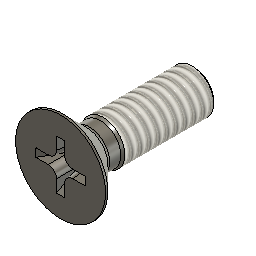
Poker Trophy (Assembly) (Autodesk Fusion 360 archive; units mm, degrees)
design "Countersunk Screw JIS B 1111 - M2x6 H Steel 4.6 Plain"
description: Countersunk Screw JIS B 1111 - M2x6 H
part number: CS JIS B 1111 - M2x6 - H Steel 4.6 Plain
Autodesk Fusion 360 part; units mm, degrees
sketch "Sketch1" plane through (0, 0, 0) normal (0, 1, 0) x (1, 0, 0)
  line L0 (0, -2.1) -> (-2, -2.1)
  line L1 (-2, -2.1) -> (-2, -2)
  line L2 (-2, -2) -> (-0.9, -0.9)
  line L3 (-1, -0.15) -> (-1, 3.9)
  line L4 (-1, 3.9) -> (0, 3.9)
  line L5 (0, 3.9) -> (0, -2.1)
  line L6 (-0.9, -0.3232) -> (-0.9, -0.9)
  line L7 (-1, -0.15) -> (-0.9, -0.3232)
  dimension "d9" = 2
  dimension "d11" = 4
  dimension "d71" = 1.2
  dimension "d72" = 1.8
  dimension "d89" = 4.05
  dimension "d101" = 30
  dimension "d115" = 6
  dimension "d121" = 45
  constraint perpendicular L0 L1
  constraint vertical L3
  constraint perpendicular L3 L4
  constraint perpendicular L0 L5
  constraint collinear origin L0.start L4.end
  constraint horizontal L0
  constraint coincident L2.end L6.end
  constraint coincident L6 L7.end
  constraint coincident L6.start L7.end
  constraint coincident origin L2
  measures "d71" distance of L0 L2.end
  measures "d89" distance of L4 L3.start
  measures "d101" angle of L3 L7
  measures "d115" distance of L0.start L4
  measures "d121" angle of L2 L5
revolve "Revolve1" add sketch "Sketch1" angle 360 about axis through (0, 0, -3.9) along (0, 0, 1) makes body 1
sketch "Sketch2" plane through (0, 0, 2.1) normal (0, 0, 1) x (1, 0, 0)
  line L0 (-0.1833, 0.1833) -> (-1.1, 0.1833)
  line L1 (-1.1, 0.1833) -> (-1.1, -0.1833)
  line L2 (-1.1, -0.1833) -> (-0.1833, -0.1833)
  line L3 (0.1833, -1.1) -> (0.1833, -0.1833)
  line L4 (-0.1833, -1.1) -> (0.1833, -1.1)
  line L5 (-0.1833, -0.1833) -> (-0.1833, -1.1)
  line L6 (1.1, 0.1833) -> (0.1833, 0.1833)
  line L7 (1.1, -0.1833) -> (1.1, 0.1833)
  line L8 (0.1833, -0.1833) -> (1.1, -0.1833)
  line L9 (-0.1833, 1.1) -> (-0.1833, 0.1833)
  line L10 (0.1833, 1.1) -> (-0.1833, 1.1)
  line L11 (0.1833, 0.1833) -> (0.1833, 1.1)
  dimension "d111" = 360
  dimension "d117" = 2.2
  dimension "d122" = 0.3667
  constraint horizontal L0
  constraint perpendicular L0 L1
  constraint vertical L0.start L2.end
  constraint coincident L0.start L9.end
  measures "d117" distance of L4.start L10
  measures "d122" distance of L0 L2
extrude "Extrude1" add sketch "Sketch2" against normal blind 1.01 draft -4 separate body makes body 2
draft "Draft1" angle -30 neutral plane through (0, 0, 2.1) pull (0, 0, 1) 4 faces at (1.0765, -0.0376, 1.7633) (0.0376, 1.0765, 1.7633) (-1.0765, 0.0376, 1.7633) (0.0376, -1.0765, 1.7633) on bodies 2
fillet "Fillet3" radius 0.3667 4 edges at (0.148, 0.148, 1.595) (0.148, -0.148, 1.595) (-0.148, -0.148, 1.595) (-0.148, 0.148, 1.595) on bodies 2
combine "Combine1" operation cut target body 1 tool bodies 2
thread "Thread1" "ISO Metric profile 2.0 M2x0.4 M2x0.4 6g" major diameter 1.9335 minor diameter 1.478 pitch 0.4 angle 60 resizes the face on face at (-0.9988, 0.0498, -1.2) on bodies 1
fillet "Fillet5" radius 0.2 1 edges at (-0.8391, 0.3255, 0.9) on bodies 1
sketch "Sketch6" plane through (0, 0, 0) normal (0, 1, 0) x (1, 0, 0)
  line L0 (-0.8, 3.9) -> (-1.02, 3.9)
  line L1 (-1.02, 3.9) -> (-1.02, 3.7)
  line L2 (-1.02, 3.7) -> (-0.8, 3.9)
  line L3 (-1, 3.9) -> (0, 3.9)
  line L4 (0, 0) -> (0, 3.9) construction
  dimension "d102" = 1.02
  dimension "d118" = 0.8
  dimension "d119" = 0.2
  constraint horizontal L0
  constraint perpendicular L0 L1
  constraint coincident L0.start L3
  constraint coincident L4.start origin
  constraint coincident L3.end L4.end
  measures "d102" distance of L4.start L1
  measures "d118" distance of L0.start L4
  measures "d119" distance of L0 L1.end
revolve "Revolve3" cut sketch "Sketch6" angle 360 about axis through (0, 0, 1.75) along (0, 0, 1) bodies 1
equation "d9 = adsk_nomdia"
equation "d11 = adsk_headdia"
equation "adsk_nomlen = 6.00 mm"
equation "adsk_headh = 1.20 mm"
equation "adsk_headdia = 4.00 mm"
equation "adsk_nomdia = 2.00 mm"
equation "adsk_headang = 90.00 deg"
equation "adsk_phildia = 2.20 mm"
equation "d31 = -adsk_phildepth"
equation "adsk_philwidth = adsk_phildia / 6"
equation "adsk_phildepth = 1.01 mm"
equation "d71 = adsk_headh"
equation "d72 = adsk_shnkdia"
equation "adsk_shnkdia = adsk_nomdia - 0.5 * adsk_pitch1"
equation "d89 = adsk_thrlen"
equation "adsk_thrlen = 4.05 mm"
equation "adsk_pitch1 = 0.40 mm"
equation "adsk_startlen = adsk_nomdia * 0.1"
equation "adsk_midfillet = 0.20 mm"
equation "d96 = adsk_midfillet"
equation "d99 = ( adsk_shnkdia / 2 ) * tan(90 deg - adsk_headang / 2) + adsk_headh"
equation "d102 = adsk_nomdia * 0.51"
equation "adsk_endpointdia = adsk_nomdia - adsk_startlen * 2"
equation "d114 = adsk_philwidth"
equation "d115 = adsk_nomlen"
equation "d117 = adsk_phildia"
equation "d118 = adsk_endpointdia / 2"
equation "d119 = adsk_startlen"
equation "d121 = adsk_headang * 0.5"
equation "d122 = adsk_philwidth"

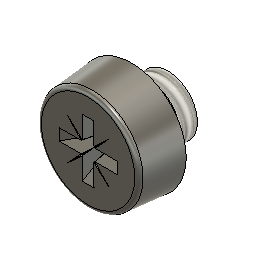
design "Cheese Head Screw SS-EN ISO 7048 - M2.5 x 1.5 - Z Steel 4.6 Plain"
description: Cheese Head Screw SS-EN ISO 7048 - M2.5 x 1.5 - Z
part number: SS-EN ISO 7048 - Z - M2.5 x 1.5 Steel 4.6 Plain
Autodesk Fusion 360 part; units mm, degrees
sketch "Sketch1" plane through (0, 0, 0) normal (0, 1, 0) x (1, 0, 0)
  line L0 (0, -1.8) -> (0, 1.5)
  line L1 (-2.25, 0) -> (-2.0925, -1.8)
  line L2 (-2.25, 0) -> (-1.0925, 0)
  line L3 (0, 1.5) -> (-1.25, 1.5)
  line L4 (-1.25, 1.5) -> (-1.25, 0.9)
  line L5 (-1.25, 0.9) -> (-1.0925, 0.3122)
  line L6 (-1.0925, 0.3122) -> (-1.0925, 0)
  line L7 (0, -1.8) -> (-2.0925, -1.8)
  dimension "d13" = 5
  dimension "d14" = 4.5
  dimension "d18" = 2.5
  dimension "d56" = 1.5
  dimension "d65" = 15
  dimension "d71" = 2.185
  dimension "d77" = 0.9
  dimension "d97" = 1.8
  constraint vertical L0
  constraint coincident origin L0
  constraint coincident origin L2
  constraint coincident L2.end L6.end
  constraint perpendicular L0 L7
  measures "d13" angle of L0 L1
  measures "d56" distance of L2 L3
  measures "d65" angle of L5 L6
  measures "d77" distance of L2 L4.end
  measures "d97" distance of L2 L7
revolve "Revolve1" add sketch "Sketch1" angle 360 about axis through (0, 0, 1.8) along (0, 0, -1) makes body 1
fillet "Fillet3" radius 0.18 1 edges at (-1.9509, 0.7567, 1.8) on bodies 1
fillet "Fillet2" radius 0.1 1 edges at (-1.0186, 0.3951, 0) on bodies 1
sketch "Sketch2" plane through (0, 0, 1.8) normal (0, 0, 1) x (1, 0, 0)
  line L0 (-0.288, -0.288) -> (0.288, -0.288)
  line L1 (0.288, -0.288) -> (0.288, 0.288)
  line L2 (0.288, 0.288) -> (-0.288, 0.288)
  line L3 (-0.288, 0.288) -> (-0.288, -0.288)
  dimension "d98" = 0.576
  constraint vertical L1
  measures "d98" distance of L0 L2
extrude "Extrude2" add sketch "Sketch2" against normal blind 0.88 draft -10 separate body makes body 2
sketch "Sketch3" plane through (0, 0, 1.8) normal (0, 0, 1) x (1, 0, 0)
  circle A0 centre (0, 0) radius 1.9276
  line L0 (-0.24, 0.24) -> (-1.2, 0.24)
  line L1 (-1.2, 0.24) -> (-1.2, -0.24)
  line L2 (-1.2, -0.24) -> (-0.24, -0.24)
  line L3 (-0.24, -0.24) -> (-0.24, -1.2)
  line L4 (-0.24, -1.2) -> (0.24, -1.2)
  line L5 (0.24, -1.2) -> (0.24, -0.24)
  line L6 (0.24, -0.24) -> (1.2, -0.24)
  line L7 (1.2, -0.24) -> (1.2, 0.24)
  line L8 (1.2, 0.24) -> (0.24, 0.24)
  line L9 (0.24, 0.24) -> (0.24, 1.2)
  line L10 (0.24, 1.2) -> (-0.24, 1.2)
  line L11 (-0.24, 1.2) -> (-0.24, 0.24)
  dimension "d86" = 360
  dimension "d87" = 2.4
  dimension "d99" = 0.48
  constraint horizontal L0
  constraint vertical L0.start L2.end
  constraint coincident L0.start L11.end
  constraint perpendicular L7 L8
  measures "d87" distance of L4.end L10
  measures "d99" distance of L0 L2
extrude "Extrude3" add sketch "Sketch3" against normal blind 1.1 draft -4 separate body contours L0 L1 L2 L3 L4 L5 L6 L7 L8 L9 L10 L11 makes body 3
draft "Draft2" angle -30 neutral plane through (0, 0, 1.8) pull (0, 0, 1) 4 faces at (-0.0544, -1.1744, 1.4333) (-1.1744, 0.0544, 1.4333) (1.1744, -0.0544, 1.4333) (0.0544, 1.1744, 1.4333) on bodies 3
combine "Combine2" operation cut target body 1 tool bodies 3 2
sketch "Sketch4" plane through (0, 0, 1.8) normal (0, 0, 1) x (1, 0, 0)
  line L0 (0.288, 0.24) -> (1.2, 0.24)
  line L1 (0.24, 1.2) -> (0.24, 0.288)
  line L2 (0, 0) -> (0.8653, 0.8653) construction
  circle A0 centre (0, 0) radius 1.2238 construction
  line L3 (0.24, 0.288) -> (0.288, 0.24)
  line L4 (0.288, 0.24) -> (0.8653, 0.8653)
  line L5 (0.24, 0.288) -> (0.8653, 0.8653)
  line L6 (-0.288, -0.288) -> (-0.288, -0.24)
  line L7 (-0.288, 0.24) -> (-0.288, 0.288)
  line L8 (-0.288, 0.288) -> (-0.24, 0.288)
  line L9 (0.24, 0.288) -> (0.288, 0.288)
  line L10 (0.288, 0.288) -> (0.288, 0.24)
  line L11 (0.288, -0.24) -> (0.288, -0.288)
  line L12 (0.288, -0.288) -> (0.24, -0.288)
  line L13 (-0.24, -0.288) -> (-0.288, -0.288)
  point P0 (0.288, 0.288)
  constraint coincident L2.start A0.centre
  constraint coincident L1.start A0
  constraint coincident L2.end A0
  constraint coincident L1.end L3.start
  constraint coincident L0.start L3.end
  constraint coincident L2 P0
extrude "Extrude4" cut sketch "Sketch4" against normal blind 1.8 draft -30 bodies 1
pattern_circular "C-Pattern1" count 4 over 360 about axis through (0, 0, 1.75) along (0, 0, 1) of "Extrude4"
thread "Thread3" "ISO Metric profile 2.5 M2.5x0.45 M2.5x0.45 6g" major diameter 2.43 minor diameter 1.9165 pitch 0.45 angle 60 resizes the face on face at (-1.2438, -0.1245, -1.3) on bodies 1
equation "adsk_nomdia = 2.50 mm"
equation "adsk_nomlen = 1.50 mm"
equation "adsk_headdia = 4.50 mm"
equation "adsk_phildia = 2.40 mm"
equation "adsk_midfillet = 0.10 mm"
equation "adsk_phildepth = 1.10 mm"
equation "adsk_shnklen = 0.90 mm"
equation "adsk_thrang = 15 deg"
equation "adsk_headang = 5 deg"
equation "d13 = adsk_headang"
equation "d14 = adsk_headdia"
equation "d18 = adsk_nomdia"
equation "adsk_philwidth = 0.48 mm"
equation "d52 = adsk_midfillet"
equation "d56 = adsk_nomlen"
equation "d65 = adsk_thrang"
equation "adsk_headh = 1.80 mm"
equation "adsk_pitch1 = 0.45 mm"
equation "adsk_shnkdia = adsk_nomdia - 0.7 * adsk_pitch1"
equation "d71 = adsk_shnkdia"
equation "adsk_headtoprad = adsk_headh * 0.1"
equation "d76 = adsk_headtoprad"
equation "d77 = adsk_shnklen"
equation "d82 = -adsk_phildepth * 0.8"
equation "d87 = adsk_phildia"
equation "d88 = -adsk_phildepth"
equation "d93 = -adsk_headh"
equation "d97 = adsk_headh"
equation "d98 = adsk_philwidth * 1.2"
equation "d99 = adsk_philwidth"
